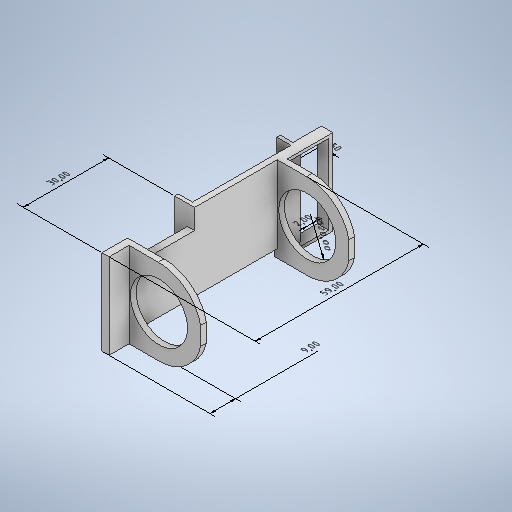
# Autodesk Inventor part: Part4-2option
Saved by Autodesk Inventor 2025.3 (Build 293356000, 356)
## iProperties
Created: 2025-08-15
Part Number: Part4-2option
Material: Generic
Document SubType Name: Modeling
Designer: Repete
Density: 1 g/cm^3
Appearance: Default
Author: Repete
Autodesk Inventor part; units mm, degrees
ref_plane "YZ Plane" through (0, 0, 0) normal (1, 0, 0) x (0, 1, 0)
ref_plane "XZ Plane" through (0, 0, 0) normal (0, 1, 0) x (-1, 0, 0)
ref_plane "XY Plane" through (0, 0, 0) normal (0, 0, 1) x (1, 0, 0)
sketch "Sketch1" plane through (0, 0, 0) normal (0, 1, 0) x (-1, 0, 0)
  line L0 (13, 14.9495) -> (0, 14.9495)
  line L1 (0, -14.9505) -> (13, -14.9505)
  line L2 (13, -14.9505) -> (13, 14.9495)
  arc A0 (-14.7414, -2.4918) -> (0, -14.9505) centre (0, 0) ccw
  arc A1 (0.2506, 14.9495) -> (-14.7414, -2.4918) centre (-0.0002, 0.001) ccw
  point P0 (13, -0.0005)
  dimension "d0" = 29.9
  dimension "d1" = 0
  dimension "d2" = 0
  constraints: 6 end point, 4 point on circle, 2 centre point, 1 horizontal, 1 midpoint, 1 parallel, 1 point on line
  measures "d0" distance of L1.end L0.start
  measures "d1" distance of point (0, 0) A0.centre
  measures "d2" distance of point (0, 0) A0.centre
extrude "Extrusion1" add sketch "Sketch1" against normal blind 60
sketch "Sketch2" plane through (0, -60, 0) normal (0, -1, 0) x (1, 0, 0)
  circle A0 centre (0, 0) radius 10
  dimension "d5" = 20
  constraints: 1 centre point, 1 coincident
  measures "d5" diameter of A0
extrude "Extrusion2" cut sketch "Sketch2" against normal through all
sketch "Sketch3" plane through (0, 0, 0) normal (0, 1, 0) x (1, 0, 0)
  line L0 (-13, -14.9495) -> (-13, 14.9505) projected
  line L1 (-0.2506, -14.9495) -> (-13, -14.9495) projected
  line L2 (-13, 14.9505) -> (-10.5, 14.9505)
  line L3 (-10.5, 14.9505) -> (-10.5, -14.9495)
  line L4 (-10.5, -14.9495) -> (-13, -14.9495)
  line L5 (-13, -14.9495) -> (-13, 14.9505)
  point P0 (0, 0)
  point P1 (0, -15)
  dimension "d8" = 2.5
  constraints: 8 end point, 2 parallel, 1 horizontal, 1 perpendicular, 2 other
  measures "d8" distance between parallel lines of L0 L3
extrude "Extrusion3" add sketch "Sketch3" against normal blind 67
sketch "Sketch4" plane through (-10.5, -67, 14.9495) normal (1, 0, 0) x (0, 0, -1)
  line L0 (-3.796, 59) -> (37.1499, 59)
  line L1 (37.1499, 59) -> (37.1499, 9)
  line L2 (37.1499, 9) -> (-3.796, 9)
  line L3 (-3.796, 9) -> (-3.796, 59)
  line L4 (29.9, 67) -> (0, 67) projected
  line L5 (0, 7) -> (29.9, 7) projected
  point P0 (14.9495, 67)
  dimension "d31" = 2
  dimension "d44" = 50
  constraints: 8 end point, 2 parallel, 1 horizontal, 1 perpendicular
  measures "d31" distance between parallel lines of L5 L2
  measures "d44" distance between parallel lines of L2 L0
extrude "Extrusion4" cut sketch "Sketch4" along normal through all
sketch "Sketch5" plane through (0, 0, 0) normal (0, 1, 0) x (1, 0, 0)
  line L0 (-13, 14.9505) -> (-13, -14.9495) projected
  line L1 (-10.5, 14.9505) -> (0, 14.9505) projected
  line L2 (-13, -14.9495) -> (-9, -14.9495)
  line L3 (-9, -14.9495) -> (-9, 14.9505)
  line L4 (-9, 14.9505) -> (-13, 14.9505)
  line L5 (-13, 14.9505) -> (-13, -14.9495)
  point P0 (0, 0)
  dimension "d13" = 4
  constraints: 8 end point, 2 parallel, 1 horizontal, 1 perpendicular, 1 point on line
  measures "d13" distance of L4.end L3.end
extrude "Extrusion5" add sketch "Sketch5" along normal blind 10
sketch "Sketch6" plane through (-9, 0, 4.3589) normal (1, 0, 0) x (0, 0, -1)
  line L0 (0, 0) -> (-10.5906, 0) projected
  line L1 (-9.5906, 0) -> (18.3094, 0)
  line L2 (18.3094, 0) -> (18.3094, 8.5)
  line L3 (18.3094, 8.5) -> (-9.5906, 8.5)
  line L4 (-9.5906, 8.5) -> (-9.5906, 0)
  line L5 (19.3094, 0) -> (19.3094, 10) projected
  line L6 (-10.5906, 0) -> (-10.5906, 10) projected
  line L7 (-10.5906, 10) -> (19.3094, 10) projected
  point P0 (4.3589, 0)
  point P1 (19.3094, 5)
  dimension "d35" = 1
  dimension "d36" = 1
  dimension "d37" = 1.5
  constraints: 8 end point, 2 parallel, 1 horizontal, 1 midpoint, 1 perpendicular, 1 point on line
  measures "d35" distance from line of point (19.309, 5) L2
  measures "d36" distance between parallel lines of L6 L4
  measures "d37" distance between parallel lines of L7 L3
extrude "Extrusion6" cut sketch "Sketch6" against normal through all
sketch "Sketch7" plane through (-13, -67, -14.9505) normal (-1, 0, 0) x (0, 0, 1)
  line L0 (29.9, 67) -> (2.9, 67)
  line L1 (2.9, 67) -> (2.9, 30)
  line L2 (2.9, 30) -> (29.9, 30)
  line L3 (29.9, 30) -> (29.9, 67)
  line L4 (28.9, 67) -> (1, 67) projected
  line L5 (29.9, 0) -> (29.9, 77) projected
  line L6 (0, 0) -> (0, 77) projected
  point P0 (14.9505, 67)
  dimension "d54" = 37
  dimension "d55" = 27
  dimension "d57" = 0
  dimension "d60" = 0
  constraints: 8 end point, 2 parallel, 1 horizontal, 1 perpendicular
  measures "d54" distance between parallel lines of L0 L2
  measures "d55" distance between parallel lines of L1 L3
  measures "d57" distance between parallel lines of L0 L4
  measures "d60" distance between parallel lines of L5 L3
extrude "Extrusion7" add sketch "Sketch7" along normal blind 4.5
sketch "Sketch8" plane through (-17.5, -67, -14.9505) normal (-1, 0, 0) x (0, 0, 1)
  line L0 (4.4, 65.75) -> (29.9, 65.75)
  line L1 (29.9, 65.75) -> (29.9, 31.25)
  line L2 (29.9, 31.25) -> (4.4, 31.25)
  line L3 (4.4, 31.25) -> (4.4, 65.75)
  line L4 (29.9, 30) -> (29.9, 67) projected
  line L5 (2.9, 30) -> (29.9, 30) projected
  point P0 (14.9505, 67)
  dimension "d61" = 0
  dimension "d62" = 34.5
  dimension "d63" = 25.5
  dimension "d64" = 1.25
  constraints: 8 end point, 2 parallel, 1 horizontal, 1 perpendicular
  measures "d61" distance between parallel lines of L4 L1
  measures "d62" distance between parallel lines of L0 L2
  measures "d63" distance between parallel lines of L1 L3
  measures "d64" distance between parallel lines of L5 L2
extrude "Extrusion8" cut sketch "Sketch8" against normal blind 5
sketch "Sketch10" plane through (-10.5, -67, 14.9495) normal (1, 0, 0) x (0, 0, -1)
  line L0 (1, 67) -> (28.9, 67)
  line L1 (28.9, 67) -> (28.9, 61)
  line L2 (28.9, 61) -> (1, 61)
  line L3 (1, 61) -> (1, 67)
  line L4 (30, 59) -> (0, 59) projected
  line L5 (29.9, 67) -> (29.9, 77) projected
  line L6 (0, 67) -> (0, 77) projected
  point P0 (14.9495, 67)
  point P1 (1, 64)
  dimension "d45" = 2
  dimension "d46" = 6
  dimension "d48" = 1
  dimension "d50" = 1
  constraints: 8 end point, 2 parallel, 1 horizontal, 1 midpoint, 1 perpendicular
  measures "d45" distance between parallel lines of L4 L2
  measures "d46" distance between parallel lines of L2 L0
  measures "d48" distance between parallel lines of L5 L1
  measures "d50" distance between parallel lines of L6 L3
extrude "Extrusion10" cut sketch "Sketch10" along normal through all
sketch "Sketch11" plane through (-9, 0, -14.9505) normal (1, 0, 0) x (0, 0, -1)
  line L0 (0, -67) -> (0, 10) projected
  line L1 (-30, 0) -> (-30, -8) projected
  line L2 (0, 1.2785) -> (-30, 1.2785)
  line L3 (-30, 1.2785) -> (-30, -6)
  line L4 (-30, -6) -> (0, -6)
  line L5 (0, -6) -> (0, 1.2785)
  line L6 (0, -8) -> (-30, -8) projected
  point P0 (-14.9505, 0)
  point P1 (0, -6)
  dimension "d51" = 2
  constraints: 8 end point, 2 parallel, 2 point on line, 1 horizontal, 1 perpendicular
  measures "d51" distance between parallel lines of L6 L4
extrude "Extrusion11" cut sketch "Sketch11" along normal through all contours L4 L1 L3 L2 L0
sketch "Sketch12" plane through (-17.5, -67, -14.9505) normal (-1, 0, 0) x (0, 0, 1)
  line L0 (2.9, 30) -> (2.9, 67) projected
  line L1 (2.9, 67) -> (20.4, 67)
  line L2 (20.4, 67) -> (20.4, 40.75)
  line L3 (20.4, 40.75) -> (2.9, 40.75)
  line L4 (2.9, 40.75) -> (2.9, 67)
  line L5 (4.4, 31.25) -> (4.4, 65.75) projected
  line L6 (4.4, 65.75) -> (29.9, 65.75) projected
  point P0 (14.9505, 67)
  point P1 (2.9, 40.75)
  dimension "d67" = 16
  dimension "d68" = 25
  constraints: 8 end point, 2 parallel, 1 horizontal, 1 perpendicular
  measures "d67" distance between parallel lines of L5 L2
  measures "d68" distance between parallel lines of L6 L3
extrude "Extrusion12" add sketch "Sketch12" against normal blind 1
sketch "Sketch13" plane through (-13, -35.75, 14.9495) normal (-1, 0, 0) x (0, 0, 1)
  line L0 (0, 0) -> (-25.5, 0) projected
  line L1 (0, 0) -> (-7, 0)
  line L2 (-7, 0) -> (-7, 13)
  line L3 (-7, 13) -> (0, 13)
  line L4 (0, 13) -> (0, 0)
  point P0 (-14.9495, 35.75)
  dimension "d76" = 7
  dimension "d77" = 13
  constraints: 8 end point, 2 parallel, 1 horizontal, 1 perpendicular
  measures "d76" distance between parallel lines of L4 L2
  measures "d77" distance between parallel lines of L0 L3
extrude "Extrusion13" [suppressed]
sketch "Sketch14" plane through (-17.5, -67, -14.9505) normal (-1, 0, 0) x (0, 0, 1)
  line L0 (7.9, 67) -> (2.9, 67)
  line L1 (2.9, 67) -> (2.9, 51)
  line L2 (2.9, 51) -> (7.9, 51)
  line L3 (7.9, 51) -> (7.9, 67)
  line L4 (2.9, 67) -> (2.9, 30) projected
  line L5 (29.9, 67) -> (2.9, 67) projected
  point P0 (14.9505, 67)
  dimension "d73" = 16
  dimension "d74" = 0
  dimension "d75" = 5
  dimension "d113" = 0
  constraints: 8 end point, 2 parallel, 1 horizontal, 1 perpendicular
  measures "d73" distance between parallel lines of L0 L2
  measures "d74" distance between parallel lines of L4 L1
  measures "d75" distance between parallel lines of L1 L3
  measures "d113" distance between parallel lines of L5 L0
extrude "Extrusion14" cut sketch "Sketch14" against normal up to surface (4.5 mm away)
sketch "Sketch15" plane through (-13, -67, -14.9505) normal (-1, 0, 0) x (0, 0, 1)
  line L0 (29.9, 9) -> (0, 9) projected
  line L1 (0, 59) -> (2.9, 59)
  line L2 (2.9, 59) -> (2.9, 9)
  line L3 (2.9, 9) -> (0, 9)
  line L4 (0, 9) -> (0, 59)
  line L5 (2.9, 51) -> (2.9, 30) projected
  line L6 (0, 0) -> (0, 77) projected
  point P0 (14.9505, 67)
  dimension "d90" = 0
  dimension "d91" = 0
  constraints: 8 end point, 2 parallel, 1 horizontal, 1 perpendicular, 1 point on line
  measures "d90" distance between parallel lines of L5 L2
  measures "d91" distance between parallel lines of L6 L4
extrude "Extrusion15" cut sketch "Sketch15" against normal through all
sketch "Sketch16" plane through (-13, -67, -14.9505) normal (-1, 0, 0) x (0, 0, 1)
  line L0 (29.9, 30) -> (2.9, 30) projected
  line L1 (29.9, 9) -> (22.9, 9)
  line L2 (22.9, 9) -> (22.9, 30)
  line L3 (22.9, 30) -> (29.9, 30)
  line L4 (29.9, 30) -> (29.9, 9)
  line L5 (29.9, 0) -> (29.9, 30) projected
  point P0 (14.9505, 67)
  dimension "d82" = 0
  dimension "d83" = 7
  constraints: 8 end point, 2 parallel, 1 horizontal, 1 perpendicular, 1 point on line
  measures "d82" distance between parallel lines of L5 L4
  measures "d83" distance between parallel lines of L4 L2
extrude "Extrusion16" cut sketch "Sketch16" against normal through all
sketch "Sketch18" plane through (-10.5, -6, 13.9495) normal (0, 1, 0) x (1, 0, 0)
  line L0 (26.137, 9.211) -> (25.1, 9.211)
  line L1 (25.1, 9.211) -> (25.1, 19.211)
  line L2 (25.1, 19.211) -> (26.137, 19.211)
  line L3 (26.137, 19.211) -> (26.137, 9.211)
  arc A0 (10.5, -1) -> (10.5, 29) centre (10.5, 14) ccw projected
  point P0 (10.5, 13.9495)
  point P1 (25.1, 14.211)
  point P2 (25.5, 14)
  point P3 (25.6185, 19.211)
  point P4 (25.6185, 9.211)
  dimension "d88" = 10
  dimension "d89" = 14.6
  constraints: 8 end point, 3 midpoint, 2 parallel, 1 horizontal, 1 perpendicular, 1 point on circle
  measures "d88" distance of point (25.618, 19.211) point (25.618, 9.211)
  measures "d89" distance from line of L1 point (10.5, 13.949)
extrude "Extrusion17" cut sketch "Sketch18" against normal through all
sketch "Sketch19" plane through (-13, -8, -14.9505) normal (-1, 0, 0) x (0, 0, 1)
  line L0 (20.4, 6.75) -> (29.9, 6.75) projected
  line L1 (-1.6421, -7.2479) -> (7.9, -7.2479)
  line L2 (7.9, -7.2479) -> (7.9, 6.75)
  line L3 (7.9, 6.75) -> (-1.6421, 6.75)
  line L4 (-1.6421, 6.75) -> (-1.6421, -7.2479)
  point P0 (14.9505, 8)
  point P1 (2.9, 6.75)
  point P2 (2.9, 6.75)
  constraints: 8 end point, 2 parallel, 1 horizontal, 1 perpendicular
extrude "Extrusion18" cut sketch "Sketch19" against normal blind 1.5
body "Solid1"
